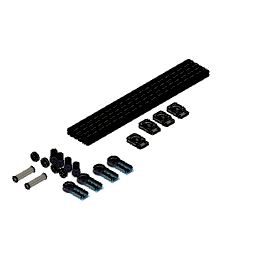
Conveyer Assemble v6 (Autodesk Fusion 360 design; units mm, degrees)
Autodesk Fusion 360 part; units mm, degrees
sketch "Sketch1" plane through (0, 0, 0) normal (0, 0, 1) x (1, 0, 0) in component "conveyerarm v2"
  line L0 (13.2288, 15) -> (80.2288, 15)
  line L1 (80.2288, 15) -> (80.2288, -15)
  line L2 (80.2288, -15) -> (13.2288, -15)
  arc A0 (13.2288, 15) -> (13.2288, -15) centre (0, 0) ccw
  dimension "d1" = 40
  dimension "d25" = 67
  constraint coincident A0.centre origin
  constraint horizontal L0
  constraint vertical L1
  constraint horizontal L2
  measures "d1" diameter of A0
  measures "d25" distance of L0.end L0.start
extrude "Extrude1" add sketch "Sketch1" along normal blind 14 makes body 1 in component "conveyerarm v2"
sketch "Sketch4" plane through (0, 0, 14) normal (0, 0, 1) x (-1, 0, 0) in component "conveyerarm v2"
  line L0 (-80.2288, -15) -> (-13.2288, -15)
  arc A0 (-13.2288, -15) -> (-13.2288, 15) centre (0, 0) ccw
  line L1 (-13.2288, 15) -> (-80.2288, 15)
  line L2 (-80.2288, 15) -> (-80.2288, -15)
  arc A1 (-12.49, -10) -> (-12.49, 10) centre (0, 0) ccw
  line L3 (-80.2288, -10) -> (-13.2288, -10)
  line L4 (-66, -10) -> (-12.49, -10)
  line L5 (-12.49, 10) -> (-80.2288, 10)
  dimension "d9" = -5
  constraint concentric A0 A1
  constraint coincident L2 L5.end
extrude "Extrude2" cut sketch "Sketch4" against normal blind 6.5 contours L2 A1 L3 L4 L5 bodies 1 in component "conveyerarm v2"
sketch "Sketch5" plane through (0, 0, 7.5) normal (0, 0, 1) x (-1, 0, 0) in component "conveyerarm v2"
  line L0 (-12.49, 10) -> (-80.2288, 10)
  line L1 (-80.2288, 10) -> (-80.2288, -10)
  line L2 (-80.2288, -10) -> (-12.49, -10)
  arc A0 (-12.49, -10) -> (-12.49, 10) centre (0, 0) ccw
  circle A1 centre (0, 0) radius 16
  dimension "d13" = 32
  constraint concentric A0 A1
  measures "d13" diameter of A1
extrude "Extrude3" cut sketch "Sketch5" against normal blind 3.5 contours A0 A1 bodies 1 in component "conveyerarm v2"
sketch "Sketch6" plane through (0, 0, 4) normal (0, 0, 1) x (-1, 0, 0) in component "conveyerarm v2"
  circle A0 centre (0, 0) radius 16
  circle A1 centre (0, 0) radius 12
  dimension "d16" = 24
  constraint coincident A0.centre A1.centre
  measures "d16" diameter of A1
extrude "Extrude4" cut sketch "Sketch6" against normal blind 5 contours A1 bodies 1 in component "conveyerarm v2"
sketch "Sketch7" plane through (0, 0, 7.5) normal (0, 0, 1) x (-1, 0, 0) in component "conveyerarm v2"
  arc A0 (-12.49, 10) -> (-12.49, -10) centre (0, 0) ccw
  line L0 (-12.49, 10) -> (-80.2288, 10)
  line L1 (-80.2288, 10) -> (-80.2288, -10)
  line L2 (-80.2288, -10) -> (-12.49, -10)
  circle A1 centre (-70.7288, 0) radius 2.6
  circle A2 centre (-48.7288, 0) radius 2.6
  circle A3 centre (-32.2288, 0) radius 2.6
  dimension "d20" = 5.2
  dimension "d21" = 22
  dimension "d22" = 5.2
  dimension "d23" = 16.5
  dimension "d24" = 5.2
  measures "d20" diameter of A1
  measures "d21" distance of A1.centre A2.centre
  measures "d22" diameter of A2
  measures "d23" distance of A2.centre A3.centre
  measures "d24" diameter of A3
extrude "Extrude5" cut sketch "Sketch7" against normal through all contours A1 | A2 | A3 bodies 1 in component "conveyerarm v2"
fillet "Fillet1" radius 5 2 edges at (80.2288, -15, 7) (80.2288, 15, 7) on bodies 1 in component "conveyerarm v2"
sketch "Sketch1 (2)" plane through (0, 0, 0) normal (0, 0, 1) x (1, 0, 0) in component "ConveyerLeg1 v3"
  line L0 (0, 0) -> (70, 0)
  line L1 (70, 0) -> (70, 42)
  line L2 (70, 42) -> (0, 42)
  line L3 (0, 42) -> (0, 0)
  dimension "d1_1" = 70
  dimension "d2" = 42
  constraint horizontal L0
  constraint vertical L1
  constraint horizontal L2
  constraint vertical L3
  constraint coincident L0.start L3.end
  measures "d1_1" distance of L1.end L2.end
  measures "d2" distance of L0.end L1.end
extrude "Extrude1'" add sketch "Sketch1 (2)" along normal blind 5 separate body makes body 2 in component "ConveyerLeg1 v3"
sketch "Sketch2" plane through (0, 0, 5) normal (0, 0, 1) x (-1, 0, 0) in component "ConveyerLeg1 v3"
  line L0 (0, -42) -> (0, 0)
  line L1 (0, 0) -> (-70, 0)
  line L2 (-70, 0) -> (-70, -42)
  line L3 (-70, -42) -> (0, -42)
  line L4 (0, 0) -> (-50, 0)
  line L5 (-50, 0) -> (-50, -42)
  line L6 (-50, -42) -> (0, -42)
  line L7 (0, -42) -> (0, 0)
  dimension "d5" = 50
  constraint horizontal L4
  constraint vertical L5
  constraint horizontal L6
  constraint vertical L7
  constraint coincident L0.end L1.start
  measures "d5" distance of L0.end L4.end
extrude "Extrude2'" add sketch "Sketch2" along normal blind 7.5 contours L0 L1 L3 L4 L5 L6 L7 bodies 2 in component "ConveyerLeg1 v3"
sketch "Sketch3" plane through (0, 0, 12.5) normal (0, 0, 1) x (-1, 0, 0) in component "ConveyerLeg1 v3"
  line L0 (0, -42) -> (0, 0)
  line L1 (0, 0) -> (-50, 0)
  line L2 (-50, 0) -> (-50, -42)
  line L3 (-50, -42) -> (0, -42)
  circle A0 centre (-25, -21) radius 18.75
  dimension "d8" = 37.5
  measures "d8" diameter of A0
hole "Hole1" at (25, 21, 12.5) direction (0, 0, -1) diameter 37.5 depth 10 tip angle 180 bodies 2 in component "ConveyerLeg1 v3"
sketch "Sketch7 (2)" plane through (0, 0, 12.5) normal (0, 0, 1) x (1, 0, 0) in component "ConveyerLeg1 v3"
  circle A0 centre (18, 21) radius 6.1
  circle A1 centre (11.3601, 28.875) radius 1.6
  circle A2 centre (25, 5.25) radius 1.6
  circle A3 centre (38.6399, 28.875) radius 1.6
  circle A4 centre (25, 36.75) radius 1.6
  circle A5 centre (25, 21) radius 18.75
  line L0 (0, 42) -> (0, 0)
  line L1 (0, 0) -> (50, 0)
  line L2 (50, 0) -> (50, 42)
  line L3 (50, 42) -> (0, 42)
  point P0 (25, 21)
  dimension "d16_1" = 3.2
  dimension "d17_1" = 3.2
  dimension "d18_1" = 3.2
  dimension "d19" = 3.2
  dimension "d41" = 12.2
  measures "d16_1" diameter of A1
  measures "d17_1" diameter of A2
  measures "d18_1" diameter of A3
  measures "d19" diameter of A4
  measures "d41" diameter of A0
extrude "Extrude3'" cut sketch "Sketch7 (2)" against normal through all contours A0 bodies 2 in component "ConveyerLeg1 v3"
extrude "Extrude4'" cut sketch "Sketch7 (2)" against normal through all contours A4 bodies 2 in component "ConveyerLeg1 v3"
extrude "Extrude5'" cut sketch "Sketch7 (2)" along normal through all and the other way through all contours A3 bodies 2 in component "ConveyerLeg1 v3"
extrude "Extrude6" cut sketch "Sketch7 (2)" along normal through all and the other way through all contours A2 bodies 2 in component "ConveyerLeg1 v3"
extrude "Extrude7" cut sketch "Sketch7 (2)" along normal through all and the other way through all contours A1 bodies 2 in component "ConveyerLeg1 v3"
sketch "Sketch9" plane through (0, 0, 5) normal (0, 0, 1) x (-1, 0, 0) in component "ConveyerLeg1 v3"
  circle A0 centre (-60, -35) radius 2.65
  circle A1 centre (-60, -7) radius 2.65
  dimension "d25_1" = 5.3
  dimension "d26_1" = 5.3
  measures "d25_1" diameter of A0
  measures "d26_1" diameter of A1
extrude "Extrude8" cut sketch "Sketch9" along normal mid plane 20 contours A0 bodies 2 in component "ConveyerLeg1 v3"
extrude "Extrude9" cut sketch "Sketch9" against normal blind 10 contours A1 bodies 2 in component "ConveyerLeg1 v3"
fillet "Fillet1'" radius 5 1 edges at (70, 42, 2.5) on bodies 2 in component "ConveyerLeg1 v3"
fillet "Fillet2" radius 5 1 edges at (70, 0, 2.5) on bodies 2 in component "ConveyerLeg1 v3"
fillet "Fillet3" radius 5 2 edges at (0, 0, 6.25) (0, 42, 6.25) on bodies 2 in component "ConveyerLeg1 v3"
sketch "Sketch10" plane through (0, 0, 12.5) normal (0, 0, 1) x (-1, 0, 0) in component "ConveyerLeg1 v3"
  circle A0 centre (-11.3598, -13.1248) radius 1.55
  circle A1 centre (-38.6402, -13.1248) radius 1.55
  point P0 (-25, -21)
  dimension "d37" = 3.1
  dimension "d38" = 3.1
  measures "d37" diameter of A0
  measures "d38" diameter of A1
extrude "Extrude10" cut sketch "Sketch10" along normal through all and the other way through all contours A1 bodies 2 in component "ConveyerLeg1 v3"
extrude "Extrude11" cut sketch "Sketch10" along normal through all and the other way through all contours A0 bodies 2 in component "ConveyerLeg1 v3"
sketch "Sketch11" plane through (0, 0, 0) normal (0, 0, 1) x (1, 0, 0) in component "ConveyerLeg1 v3"
sketch "Sketch1 (3)" plane through (0, 0, 0) normal (0, 0, 1) x (1, 0, 0) in component "CONVEYERROLLERv2 v4"
  circle A0 centre (0, 0) radius 9.95
  dimension "d1_3" = 19.9
  constraint coincident A0.centre origin
  measures "d1_3" diameter of A0
extrude "Extrude1''" add sketch "Sketch1 (3)" along normal blind 40 separate body makes body 3 in component "CONVEYERROLLERv2 v4"
sketch "Sketch2 (2)" plane through (0, 0, 0) normal (1, 0, 0) x (0, 1, 0) in component "CONVEYERROLLERv2 v4"
  line L0 (-12, 12) -> (-9.9, 9.9)
  line L1 (-12, 12) -> (-9.9, 14.1)
  line L2 (-9.9, 9.9) -> (-9.9, 14.1)
  constraint perpendicular L0 L1
revolve "Revolve1" add sketch "Sketch2 (2)" angle 360 about axis through (0, 0, 0) along (0, 0, -1) separate body makes body 4 in component "CONVEYERROLLERv2 v4"
sketch "Sketch4 (2)" plane through (0, 0, 40) normal (0, 0, 1) x (-1, 0, 0) in component "CONVEYERROLLERv2 v4"
  line L0 (-9.4994, -0.1031) -> (-9.4994, -0.1031)
  circle A0 centre (0, 0) radius 8.5
  circle A1 centre (0, 0) radius 10
  dimension "d32_2" = 17
  dimension "d33_2" = 20
  constraint coincident A0.centre A1.centre
  constraint concentric A0 A1
  measures "d32_2" diameter of A0
  measures "d33_2" diameter of A1
extrude "Extrude6'" cut sketch "Sketch4 (2)" against normal blind 18 bodies 3 in component "CONVEYERROLLERv2 v4"
sketch "Sketch9 (2)" plane through (0, 0, 40) normal (0, 0, 1) x (-1, 0, 0) in component "CONVEYERROLLERv2 v4"
  circle A0 centre (0, 0) radius 8.5
  line L0 (7.1105, -6.3018) -> (6.4494, -5.5367)
  line L1 (5.8562, -6.1607) -> (6.6539, -6.7822)
  line L2 (7.1105, -6.3018) -> (6.6539, -6.7822)
  line L3 (5.8562, -6.1607) -> (6.4494, -5.5367)
  line L4 (6.9765, -4.8558) -> (7.8829, -5.3039)
  line L5 (8.2335, -4.7415) -> (7.8829, -5.3039)
  line L6 (8.2335, -4.7415) -> (7.4319, -4.1251)
  line L7 (6.9765, -4.8558) -> (7.4319, -4.1251)
  line L8 (7.8111, -3.352) -> (8.7892, -3.6085)
  line L9 (9.0194, -2.9871) -> (8.7892, -3.6085)
  line L10 (9.0194, -2.9871) -> (8.1102, -2.5446)
  line L11 (7.8111, -3.352) -> (8.1102, -2.5446)
  line L12 (8.326, -1.711) -> (9.3357, -1.7654)
  line L13 (9.4361, -1.1103) -> (9.3357, -1.7654)
  line L14 (9.4361, -1.1103) -> (8.4564, -0.8599)
  line L15 (8.326, -1.711) -> (8.4564, -0.8599)
  line L16 (8.5, 0) -> (9.5, 0.15)
  line L17 (9.4664, 0.8119) -> (9.5, 0.15)
  line L18 (9.4664, 0.8119) -> (8.4564, 0.8599)
  line L19 (8.5, 0) -> (8.4564, 0.8599)
  line L20 (8.326, 1.711) -> (9.2753, 2.0593)
  line L21 (9.1092, 2.7008) -> (9.2753, 2.0593)
  line L22 (9.1092, 2.7008) -> (8.1102, 2.5446)
  line L23 (8.326, 1.711) -> (8.1102, 2.5446)
  line L24 (7.8111, 3.352) -> (8.6709, 3.8842)
  line L25 (8.3791, 4.4792) -> (8.6709, 3.8842)
  line L26 (8.3791, 4.4792) -> (7.4319, 4.1251)
  line L27 (7.8111, 3.352) -> (7.4319, 4.1251)
  line L28 (6.9765, 4.8558) -> (7.7116, 5.5502)
  line L29 (7.3059, 6.0742) -> (7.7116, 5.5502)
  line L30 (7.3059, 6.0742) -> (6.4494, 5.5367)
  line L31 (6.9765, 4.8558) -> (6.4494, 5.5367)
  line L32 (5.8562, 6.1607) -> (6.4365, 6.9889)
  line L33 (5.9336, 7.4206) -> (6.4365, 6.9889)
  line L34 (5.9336, 7.4206) -> (5.2029, 6.7216)
  line L35 (5.8562, 6.1607) -> (5.2029, 6.7216)
  line L36 (4.4962, 7.2135) -> (4.8979, 8.1415)
  line L37 (4.3184, 8.4631) -> (4.8979, 8.1415)
  line L38 (4.3184, 8.4631) -> (3.7434, 7.6313)
  line L39 (4.4962, 7.2135) -> (3.7434, 7.6313)
  line L40 (2.9521, 7.9709) -> (3.1587, 8.9607)
  line L41 (2.5264, 9.1591) -> (3.1587, 8.9607)
  line L42 (2.5264, 9.1591) -> (2.1305, 8.2287)
  line L43 (2.9521, 7.9709) -> (2.1305, 8.2287)
  line L44 (1.2871, 8.402) -> (1.2903, 9.4132)
  line L45 (0.631, 9.4802) -> (1.2903, 9.4132)
  line L46 (0.631, 9.4802) -> (0.4305, 8.4891)
  line L47 (1.2871, 8.402) -> (0.4305, 8.4891)
  line L48 (-0.4305, 8.4891) -> (-0.631, 9.4802)
  line L49 (-1.2903, 9.4132) -> (-0.631, 9.4802)
  line L50 (-1.2903, 9.4132) -> (-1.2871, 8.402)
  line L51 (-0.4305, 8.4891) -> (-1.2871, 8.402)
  line L52 (-2.1305, 8.2287) -> (-2.5264, 9.1591)
  line L53 (-3.1587, 8.9607) -> (-2.5264, 9.1591)
  line L54 (-3.1587, 8.9607) -> (-2.9521, 7.9709)
  line L55 (-2.1305, 8.2287) -> (-2.9521, 7.9709)
  line L56 (-3.7434, 7.6313) -> (-4.3184, 8.4631)
  line L57 (-4.8979, 8.1415) -> (-4.3184, 8.4631)
  line L58 (-4.8979, 8.1415) -> (-4.4962, 7.2135)
  line L59 (-3.7434, 7.6313) -> (-4.4962, 7.2135)
  line L60 (-5.2029, 6.7216) -> (-5.9336, 7.4206)
  line L61 (-6.4365, 6.9889) -> (-5.9336, 7.4206)
  line L62 (-6.4365, 6.9889) -> (-5.8562, 6.1607)
  line L63 (-5.2029, 6.7216) -> (-5.8562, 6.1607)
  line L64 (-6.4494, 5.5367) -> (-7.3059, 6.0742)
  line L65 (-7.7116, 5.5502) -> (-7.3059, 6.0742)
  line L66 (-7.7116, 5.5502) -> (-6.9765, 4.8558)
  line L67 (-6.4494, 5.5367) -> (-6.9765, 4.8558)
  line L68 (-7.4319, 4.1251) -> (-8.3791, 4.4792)
  line L69 (-8.6709, 3.8842) -> (-8.3791, 4.4792)
  line L70 (-8.6709, 3.8842) -> (-7.8111, 3.352)
  line L71 (-7.4319, 4.1251) -> (-7.8111, 3.352)
  line L72 (-8.1102, 2.5446) -> (-9.1092, 2.7008)
  line L73 (-9.2753, 2.0593) -> (-9.1092, 2.7008)
  line L74 (-9.2753, 2.0593) -> (-8.326, 1.711)
  line L75 (-8.1102, 2.5446) -> (-8.326, 1.711)
  line L76 (-8.4564, 0.8599) -> (-9.4664, 0.8119)
  line L77 (-9.5, 0.15) -> (-9.4664, 0.8119)
  line L78 (-9.5, 0.15) -> (-8.5, 0)
  line L79 (-8.4564, 0.8599) -> (-8.5, 0)
  line L80 (-8.4564, -0.8599) -> (-9.4361, -1.1103)
  line L81 (-9.3357, -1.7654) -> (-9.4361, -1.1103)
  line L82 (-9.3357, -1.7654) -> (-8.326, -1.711)
  line L83 (-8.4564, -0.8599) -> (-8.326, -1.711)
  line L84 (-8.1102, -2.5446) -> (-9.0194, -2.9871)
  line L85 (-8.7892, -3.6085) -> (-9.0194, -2.9871)
  line L86 (-8.7892, -3.6085) -> (-7.8111, -3.352)
  line L87 (-8.1102, -2.5446) -> (-7.8111, -3.352)
  line L88 (-7.4319, -4.1251) -> (-8.2335, -4.7415)
  line L89 (-7.8829, -5.3039) -> (-8.2335, -4.7415)
  line L90 (-7.8829, -5.3039) -> (-6.9765, -4.8558)
  line L91 (-7.4319, -4.1251) -> (-6.9765, -4.8558)
  line L92 (-6.4494, -5.5367) -> (-7.1105, -6.3018)
  line L93 (-6.6539, -6.7822) -> (-7.1105, -6.3018)
  line L94 (-6.6539, -6.7822) -> (-5.8562, -6.1607)
  line L95 (-6.4494, -5.5367) -> (-5.8562, -6.1607)
  line L96 (-5.2029, -6.7216) -> (-5.6964, -7.6042)
  line L97 (-5.1524, -7.9828) -> (-5.6964, -7.6042)
  line L98 (-5.1524, -7.9828) -> (-4.4962, -7.2135)
  line L99 (-5.2029, -6.7216) -> (-4.4962, -7.2135)
  line L100 (-3.7434, -7.6313) -> (-4.0491, -8.5952)
  line L101 (-3.4401, -8.8566) -> (-4.0491, -8.5952)
  line L102 (-3.4401, -8.8566) -> (-2.9521, -7.9709)
  line L103 (-3.7434, -7.6313) -> (-2.9521, -7.9709)
  line L104 (-2.1305, -8.2287) -> (-2.236, -9.2343)
  line L105 (-1.5868, -9.3677) -> (-2.236, -9.2343)
  line L106 (-1.5868, -9.3677) -> (-1.2871, -8.402)
  line L107 (-2.1305, -8.2287) -> (-1.2871, -8.402)
  line L108 (-0.4305, -8.4891) -> (-0.3314, -9.4954)
  line L109 (0.3314, -9.4954) -> (-0.3314, -9.4954)
  line L110 (0.3314, -9.4954) -> (0.4305, -8.4891)
  line L111 (-0.4305, -8.4891) -> (0.4305, -8.4891)
  line L112 (1.2871, -8.402) -> (1.5868, -9.3677)
  line L113 (2.236, -9.2343) -> (1.5868, -9.3677)
  line L114 (2.236, -9.2343) -> (2.1305, -8.2287)
  line L115 (1.2871, -8.402) -> (2.1305, -8.2287)
  line L116 (2.9521, -7.9709) -> (3.4401, -8.8566)
  line L117 (4.0491, -8.5952) -> (3.4401, -8.8566)
  line L118 (4.0491, -8.5952) -> (3.7434, -7.6313)
  line L119 (2.9521, -7.9709) -> (3.7434, -7.6313)
  line L120 (4.4962, -7.2135) -> (5.1524, -7.9828)
  line L121 (5.6964, -7.6042) -> (5.1524, -7.9828)
  line L122 (5.6964, -7.6042) -> (5.2029, -6.7216)
  line L123 (4.4962, -7.2135) -> (5.2029, -6.7216)
  dimension "d42_1" = 360
extrude "Extrude7'" add sketch "Sketch9 (2)" against normal blind 18 contours A0 L16 L17 L18 | A0 L12 L13 L14 | A0 L20 L21 L22 | A0 L8 L9 L10 | A0 L24 L25 L26 | A0 L4 L5 L6 | A0 L28 L29 L30 | A0 L0 L1 L2 | A0 L32 L33 L34 | A0 L120 L121 L122 | A0 L36 L37 L38 | A0 L116 L117 L118 | A0 L40 L41 L42 | A0 L112 L113 L114 | A0 L44 L45 L46 | A0 L108 L109 L110 | A0 L48 L49 L50 | A0 L104 L105 L106 | A0 L52 L53 L54 | A0 L100 L101 L102 | A0 L56 L57 L58 | A0 L96 L97 L98 | A0 L60 L61 L62 | A0 L92 L93 L94 | A0 L64 L65 L66 | A0 L88 L89 L90 | A0 L68 L69 L70 | A0 L84 L85 L86 | A0 L72 L73 L74 | A0 L80 L81 L82 | A0 L76 L77 L78 bodies 3 in component "CONVEYERROLLERv2 v4"
sketch "Sketch11 (2)" plane through (0, 0, 40) normal (0, 0, 1) x (-1, 0, 0) in component "CONVEYERROLLERv2 v4"
  arc A0 (-4.4962, -7.2135) -> (-3.7434, -7.6313) centre (0, 0) ccw
  line L0 (-3.7434, -7.6313) -> (-4.0491, -8.5952)
  line L1 (-4.0491, -8.5952) -> (-3.4401, -8.8566)
  line L2 (-3.4401, -8.8566) -> (-2.9521, -7.9709)
  arc A1 (-2.9521, -7.9709) -> (-2.1305, -8.2287) centre (0, 0) ccw
  line L3 (-2.1305, -8.2287) -> (-2.236, -9.2343)
  line L4 (-2.236, -9.2343) -> (-1.5868, -9.3677)
  line L5 (-1.5868, -9.3677) -> (-1.2871, -8.402)
  arc A2 (-1.2871, -8.402) -> (-0.4305, -8.4891) centre (0, 0) ccw
  line L6 (-0.4305, -8.4891) -> (-0.3314, -9.4954)
  line L7 (-0.3314, -9.4954) -> (0.3314, -9.4954)
  line L8 (0.3314, -9.4954) -> (0.4305, -8.4891)
  arc A3 (0.4305, -8.4891) -> (1.2871, -8.402) centre (0, 0) ccw
  line L9 (1.2871, -8.402) -> (1.5868, -9.3677)
  line L10 (1.5868, -9.3677) -> (2.236, -9.2343)
  line L11 (2.236, -9.2343) -> (2.1305, -8.2287)
  arc A4 (2.1305, -8.2287) -> (2.9521, -7.9709) centre (0, 0) ccw
  line L12 (2.9521, -7.9709) -> (3.4401, -8.8566)
  line L13 (3.4401, -8.8566) -> (4.0491, -8.5952)
  line L14 (4.0491, -8.5952) -> (3.7434, -7.6313)
  arc A5 (3.7434, -7.6313) -> (4.4962, -7.2135) centre (0, 0) ccw
  line L15 (4.4962, -7.2135) -> (5.1524, -7.9828)
  line L16 (5.1524, -7.9828) -> (5.6964, -7.6042)
  line L17 (5.6964, -7.6042) -> (5.2029, -6.7216)
  arc A6 (5.2029, -6.7216) -> (5.8562, -6.1607) centre (0, 0) ccw
  line L18 (5.8562, -6.1607) -> (6.6539, -6.7822)
  line L19 (6.6539, -6.7822) -> (7.1105, -6.3018)
  line L20 (7.1105, -6.3018) -> (6.4494, -5.5367)
  arc A7 (6.4494, -5.5367) -> (6.9765, -4.8558) centre (0, 0) ccw
  line L21 (6.9765, -4.8558) -> (7.8829, -5.3039)
  line L22 (7.8829, -5.3039) -> (8.2335, -4.7415)
  line L23 (8.2335, -4.7415) -> (7.4319, -4.1251)
  arc A8 (7.4319, -4.1251) -> (7.8111, -3.352) centre (0, 0) ccw
  line L24 (7.8111, -3.352) -> (8.7892, -3.6085)
  line L25 (8.7892, -3.6085) -> (9.0194, -2.9871)
  line L26 (9.0194, -2.9871) -> (8.1102, -2.5446)
  arc A9 (8.1102, -2.5446) -> (8.326, -1.711) centre (0, 0) ccw
  line L27 (8.326, -1.711) -> (9.3357, -1.7654)
  line L28 (9.3357, -1.7654) -> (9.4361, -1.1103)
  line L29 (9.4361, -1.1103) -> (8.4564, -0.8599)
  arc A10 (8.4564, -0.8599) -> (8.5, 0) centre (0, 0) ccw
  line L30 (8.5, 0) -> (9.5, 0.15)
  line L31 (9.5, 0.15) -> (9.4664, 0.8119)
  line L32 (9.4664, 0.8119) -> (8.4564, 0.8599)
  arc A11 (8.4564, 0.8599) -> (8.326, 1.711) centre (0, 0) ccw
  line L33 (8.326, 1.711) -> (9.2753, 2.0593)
  line L34 (9.2753, 2.0593) -> (9.1092, 2.7008)
  line L35 (9.1092, 2.7008) -> (8.1102, 2.5446)
  arc A12 (8.1102, 2.5446) -> (7.8111, 3.352) centre (0, 0) ccw
  line L36 (7.8111, 3.352) -> (8.6709, 3.8842)
  line L37 (8.6709, 3.8842) -> (8.3791, 4.4792)
  line L38 (8.3791, 4.4792) -> (7.4319, 4.1251)
  arc A13 (7.4319, 4.1251) -> (6.9765, 4.8558) centre (0, 0) ccw
  line L39 (6.9765, 4.8558) -> (7.7116, 5.5502)
  line L40 (7.7116, 5.5502) -> (7.3059, 6.0742)
  line L41 (7.3059, 6.0742) -> (6.4494, 5.5367)
  arc A14 (6.4494, 5.5367) -> (5.8562, 6.1607) centre (0, 0) ccw
  line L42 (5.8562, 6.1607) -> (6.4365, 6.9889)
  line L43 (6.4365, 6.9889) -> (5.9336, 7.4206)
  line L44 (5.9336, 7.4206) -> (5.2029, 6.7216)
  arc A15 (5.2029, 6.7216) -> (4.4962, 7.2135) centre (0, 0) ccw
  line L45 (4.4962, 7.2135) -> (4.8979, 8.1415)
  line L46 (4.8979, 8.1415) -> (4.3184, 8.4631)
  line L47 (4.3184, 8.4631) -> (3.7434, 7.6313)
  arc A16 (3.7434, 7.6313) -> (2.9521, 7.9709) centre (0, 0) ccw
  line L48 (2.9521, 7.9709) -> (3.1587, 8.9607)
  line L49 (3.1587, 8.9607) -> (2.5264, 9.1591)
  line L50 (2.5264, 9.1591) -> (2.1305, 8.2287)
  arc A17 (2.1305, 8.2287) -> (1.2871, 8.402) centre (0, 0) ccw
  line L51 (1.2871, 8.402) -> (1.2903, 9.4132)
  line L52 (1.2903, 9.4132) -> (0.631, 9.4802)
  line L53 (0.631, 9.4802) -> (0.4305, 8.4891)
  arc A18 (0.4305, 8.4891) -> (-0.4305, 8.4891) centre (0, 0) ccw
  line L54 (-0.4305, 8.4891) -> (-0.631, 9.4802)
  line L55 (-0.631, 9.4802) -> (-1.2903, 9.4132)
  line L56 (-1.2903, 9.4132) -> (-1.2871, 8.402)
  arc A19 (-1.2871, 8.402) -> (-2.1305, 8.2287) centre (0, 0) ccw
  line L57 (-2.1305, 8.2287) -> (-2.5264, 9.1591)
  line L58 (-2.5264, 9.1591) -> (-3.1587, 8.9607)
  line L59 (-3.1587, 8.9607) -> (-2.9521, 7.9709)
  arc A20 (-2.9521, 7.9709) -> (-3.7434, 7.6313) centre (0, 0) ccw
  line L60 (-3.7434, 7.6313) -> (-4.3184, 8.4631)
  line L61 (-4.3184, 8.4631) -> (-4.8979, 8.1415)
  line L62 (-4.8979, 8.1415) -> (-4.4962, 7.2135)
  arc A21 (-4.4962, 7.2135) -> (-5.2029, 6.7216) centre (0, 0) ccw
  line L63 (-5.2029, 6.7216) -> (-5.9336, 7.4206)
  line L64 (-5.9336, 7.4206) -> (-6.4365, 6.9889)
  line L65 (-6.4365, 6.9889) -> (-5.8562, 6.1607)
  arc A22 (-5.8562, 6.1607) -> (-6.4494, 5.5367) centre (0, 0) ccw
  line L66 (-6.4494, 5.5367) -> (-7.3059, 6.0742)
  line L67 (-7.3059, 6.0742) -> (-7.7116, 5.5502)
  line L68 (-7.7116, 5.5502) -> (-6.9765, 4.8558)
  arc A23 (-6.9765, 4.8558) -> (-7.4319, 4.1251) centre (0, 0) ccw
  line L69 (-7.4319, 4.1251) -> (-8.3791, 4.4792)
  line L70 (-8.3791, 4.4792) -> (-8.6709, 3.8842)
  line L71 (-8.6709, 3.8842) -> (-7.8111, 3.352)
  arc A24 (-7.8111, 3.352) -> (-8.1102, 2.5446) centre (0, 0) ccw
  line L72 (-8.1102, 2.5446) -> (-9.1092, 2.7008)
  line L73 (-9.1092, 2.7008) -> (-9.2753, 2.0593)
  line L74 (-9.2753, 2.0593) -> (-8.326, 1.711)
  arc A25 (-8.326, 1.711) -> (-8.4564, 0.8599) centre (0, 0) ccw
  line L75 (-8.4564, 0.8599) -> (-9.4664, 0.8119)
  line L76 (-9.4664, 0.8119) -> (-9.5, 0.15)
  line L77 (-9.5, 0.15) -> (-8.5, 0)
  arc A26 (-8.5, 0) -> (-8.4564, -0.8599) centre (0, 0) ccw
  line L78 (-8.4564, -0.8599) -> (-9.4361, -1.1103)
  line L79 (-9.4361, -1.1103) -> (-9.3357, -1.7654)
  line L80 (-9.3357, -1.7654) -> (-8.326, -1.711)
  arc A27 (-8.326, -1.711) -> (-8.1102, -2.5446) centre (0, 0) ccw
  line L81 (-8.1102, -2.5446) -> (-9.0194, -2.9871)
  line L82 (-9.0194, -2.9871) -> (-8.7892, -3.6085)
  line L83 (-8.7892, -3.6085) -> (-7.8111, -3.352)
  arc A28 (-7.8111, -3.352) -> (-7.4319, -4.1251) centre (0, 0) ccw
  line L84 (-7.4319, -4.1251) -> (-8.2335, -4.7415)
  line L85 (-8.2335, -4.7415) -> (-7.8829, -5.3039)
  line L86 (-7.8829, -5.3039) -> (-6.9765, -4.8558)
  arc A29 (-6.9765, -4.8558) -> (-6.4494, -5.5367) centre (0, 0) ccw
  line L87 (-6.4494, -5.5367) -> (-7.1105, -6.3018)
  line L88 (-7.1105, -6.3018) -> (-6.6539, -6.7822)
  line L89 (-6.6539, -6.7822) -> (-5.8562, -6.1607)
  arc A30 (-5.8562, -6.1607) -> (-5.2029, -6.7216) centre (0, 0) ccw
  line L90 (-5.2029, -6.7216) -> (-5.6964, -7.6042)
  line L91 (-5.6964, -7.6042) -> (-5.1524, -7.9828)
  line L92 (-5.1524, -7.9828) -> (-4.4962, -7.2135)
  circle A31 centre (0, 0) radius 4
  dimension "d45_1" = 8
  constraint concentric A0 A31
  measures "d45_1" diameter of A31
extrude "Extrude8'" cut sketch "Sketch11 (2)" against normal through all contours A31 bodies 3 in component "CONVEYERROLLERv2 v4"
fillet "Fillet1''" radius 0.1 2 edges at (4.3184, -8.4631, 31) (4.8979, -8.1415, 31) on bodies 3 in component "CONVEYERROLLERv2 v4"
fillet "Fillet2'" radius 0.1 9 edges at (3.1587, -8.9607, 31) (2.5264, -9.1591, 31) (1.2903, -9.4132, 31) (0.631, -9.4802, 31) (-0.631, -9.4802, 31) (6.4365, -6.9889, 31) (5.9336, -7.4206, 31) (7.3059, -6.0742, 31) (7.7116, -5.5502, 31) on bodies 3 in component "CONVEYERROLLERv2 v4"
fillet "Fillet3'" radius 0.1 51 edges at (8.3791, -4.4792, 31) (8.6709, -3.8842, 31) (9.1092, -2.7008, 31) (9.2753, -2.0593, 31) (9.4664, -0.8119, 31) (9.5, -0.15, 31) (9.4361, 1.1103, 31) (9.3357, 1.7654, 31) (9.0194, 2.9871, 31) (8.7892, 3.6085, 31) (8.2335, 4.7415, 31) (7.8829, 5.3039, 31) (7.1105, 6.3018, 31) (6.6539, 6.7822, 31) (5.6964, 7.6042, 31) (-9.3357, 1.7654, 31) (-9.4361, 1.1103, 31) (-9.5, -0.15, 31) (-9.4664, -0.8119, 31) (-9.2753, -2.0593, 31) (-9.1092, -2.7008, 31) (-8.6709, -3.8842, 31) (-8.3791, -4.4792, 31) (-7.7116, -5.5502, 31) (-7.3059, -6.0742, 31) (-6.4365, -6.9889, 31) (-5.9336, -7.4206, 31) (-4.8979, -8.1415, 31) (-4.3184, -8.4631, 31) (-3.1587, -8.9607, 31) (-2.5264, -9.1591, 31) (-1.2903, -9.4132, 31) (-9.0194, 2.9871, 31) (-8.7892, 3.6085, 31) (-8.2335, 4.7415, 31) (-7.8829, 5.3039, 31) (-7.1105, 6.3018, 31) (-6.6539, 6.7822, 31) (-5.6964, 7.6042, 31) (-5.1524, 7.9828, 31) (-4.0491, 8.5952, 31) (-2.236, 9.2343, 31) (-1.5868, 9.3677, 31) (-0.3314, 9.4954, 31) (0.3314, 9.4954, 31) (1.5868, 9.3677, 31) (2.236, 9.2343, 31) (3.4401, 8.8566, 31) (4.0491, 8.5952, 31) (5.1524, 7.9828, 31) (-3.4401, 8.8566, 31) on bodies 3 in component "CONVEYERROLLERv2 v4"
sketch "Sketch12" plane through (0, 0, 0) normal (0, 0, 1) x (1, 0, 0) in component "CONVEYERROLLERv2 v4"
  circle A0 centre (0, 0) radius 10.5
  circle A1 centre (0, 0) radius 8.85
  dimension "d54" = 21
  dimension "d55" = 17.7
  constraint coincident A0.centre A1.centre
  constraint concentric A0 A1
  measures "d54" diameter of A0
  measures "d55" diameter of A1
extrude "Extrude9'" cut sketch "Sketch12" along normal blind 9 bodies 3 in component "CONVEYERROLLERv2 v4"
combine "Combine4" operation add target body 3 tool bodies 4 in component "CONVEYERROLLERv2 v4"
sketch "Sketch1 (4)" plane through (0, 0, 0) normal (0, 1, 0) x (1, 0, 0) in component "ProfileBase"
  line L0 (0, 0) -> (100, 0)
  line L1 (100, 0) -> (100, -20)
  line L2 (100, -20) -> (0, -20)
  line L3 (0, -20) -> (0, 0)
  dimension "d53" = 100
  dimension "d58" = 20
  constraint horizontal L0
  constraint vertical L1
  constraint horizontal L2
  constraint vertical L3
  constraint coincident L0.start L3.end
  measures "d53" distance of L0.start L0.end
  measures "d58" distance of L0.start L2.end
extrude "Extrude1'''" add sketch "Sketch1 (4)" along normal blind 600 separate body makes body 5 in component "ProfileBase"
sketch "Sketch2 (3)" plane through (0, 0, 0) normal (0, -1, 0) x (1, 0, 0) in component "ProfileBase"
  line L0 (100, 20) -> (0, 20)
  line L1 (0, 20) -> (0, 0)
  line L2 (0, 0) -> (100, 0)
  line L3 (100, 0) -> (100, 20)
  circle A0 centre (10, 10) radius 2.5
  line L4 (0, 13) -> (2, 13)
  line L5 (2, 13) -> (2, 17)
  line L6 (2, 17) -> (6, 13)
  line L7 (6, 13) -> (6, 7)
  line L8 (6, 7) -> (2, 3)
  line L9 (2, 3) -> (2, 7)
  line L10 (2, 7) -> (0, 7)
  line L11 (0, 13) -> (0, 7)
  line L12 (3, 2) -> (7, 6)
  line L13 (7, 2) -> (3, 2)
  line L14 (7, 0) -> (7, 2)
  line L15 (7, 0) -> (13, 0)
  line L16 (13, 2) -> (13, 0)
  line L17 (17, 2) -> (13, 2)
  line L18 (13, 6) -> (17, 2)
  line L19 (7, 6) -> (13, 6)
  line L20 (18, 3) -> (14, 7)
  line L21 (18, 7) -> (18, 3)
  line L22 (20, 7) -> (18, 7)
  line L23 (20, 7) -> (20, 13)
  line L24 (18, 13) -> (20, 13)
  line L25 (18, 17) -> (18, 13)
  line L26 (14, 13) -> (18, 17)
  line L27 (14, 7) -> (14, 13)
  line L28 (17, 18) -> (13, 14)
  line L29 (13, 18) -> (17, 18)
  line L30 (13, 20) -> (13, 18)
  line L31 (13, 20) -> (7, 20)
  line L32 (7, 18) -> (7, 20)
  line L33 (3, 18) -> (7, 18)
  line L34 (7, 14) -> (3, 18)
  line L35 (13, 14) -> (7, 14)
  point P0 (6, 10)
  dimension "d61" = 5
  dimension "d62" = 10
  dimension "d63" = 10
  dimension "d64" = 4
  dimension "d65" = 6
  dimension "d66" = 2
  dimension "d67" = 2
  dimension "d69" = 3
  dimension "d70" = 6
  dimension "d71" = 3
  dimension "d72" = 90
  dimension "d74" = 360
  constraint coincident L1 L4.start
  constraint perpendicular L1 L4
  constraint perpendicular L4 L5
  constraint parallel L1 L7
  constraint parallel L7 L9
  constraint coincident L1 L10.end
  constraint perpendicular L1 L10
  constraint equal L5 L9
  constraint midpoint L7 P0
  measures "d61" diameter of A0
  measures "d62" distance of L1 A0.centre
  measures "d63" distance of L2 A0.centre
  measures "d64" distance of A0.centre L7
  measures "d65" distance of L6.end L7.end
  measures "d66" distance of L1 L5
  measures "d67" distance of L1 L9
  measures "d69" distance of A0.centre L10
  measures "d70" distance of L4 L10
  measures "d71" distance of L10 P0
  measures "d72" angle of L6 L8
extrude "Extrude2''" cut sketch "Sketch2 (3)" against normal through all contours L0 L28 L29 L30 L31 L32 L33 L34 L35 | L2 L12 L13 L14 L15 L16 L17 L18 L19 | L1 L4 L5 L6 L7 L8 L9 L10 L11 | A0 | L20 L21 L22 L23 L24 L25 L26 L27 bodies 5 in component "ProfileBase"
pattern_linear "R-Pattern1" count 5 spacing 20 along (1, 0, 0) of "Extrude2''" in component "ProfileBase"
sketch "Sketch3 (2)" plane through (0, 0, 0) normal (0, -1, 0) x (1, 0, 0) in component "ProfileBase"
  circle A0 centre (90, 10) radius 2.5
  line L0 (78, 13) -> (82, 13)
  line L1 (82, 13) -> (82, 17)
  line L2 (82, 17) -> (86, 13)
  line L3 (86, 13) -> (86, 7)
  line L4 (86, 7) -> (82, 3)
  line L5 (82, 3) -> (82, 7)
  line L6 (82, 7) -> (78, 7)
  line L7 (78, 7) -> (78, 3)
  line L8 (78, 3) -> (74, 7)
  line L9 (74, 7) -> (74, 13)
  line L10 (74, 13) -> (78, 17)
  line L11 (78, 17) -> (78, 13)
  circle A1 centre (70, 10) radius 2.5
  line L12 (58, 13) -> (62, 13)
  line L13 (62, 13) -> (62, 17)
  line L14 (62, 17) -> (66, 13)
  line L15 (66, 13) -> (66, 7)
  line L16 (66, 7) -> (62, 3)
  line L17 (62, 3) -> (62, 7)
  line L18 (62, 7) -> (58, 7)
  line L19 (58, 7) -> (58, 3)
  line L20 (58, 3) -> (54, 7)
  line L21 (54, 7) -> (54, 13)
  line L22 (54, 13) -> (58, 17)
  line L23 (58, 17) -> (58, 13)
  circle A2 centre (50, 10) radius 2.5
  line L24 (38, 13) -> (42, 13)
  line L25 (42, 13) -> (42, 17)
  line L26 (42, 17) -> (46, 13)
  line L27 (46, 13) -> (46, 7)
  line L28 (46, 7) -> (42, 3)
  line L29 (42, 3) -> (42, 7)
  line L30 (42, 7) -> (38, 7)
  line L31 (38, 7) -> (38, 3)
  line L32 (38, 3) -> (34, 7)
  line L33 (34, 7) -> (34, 13)
  line L34 (34, 13) -> (38, 17)
  line L35 (38, 17) -> (38, 13)
  circle A3 centre (30, 10) radius 2.5
  line L36 (100, 7) -> (98, 7)
  line L37 (98, 7) -> (98, 3)
  line L38 (98, 3) -> (94, 7)
  line L39 (94, 7) -> (94, 13)
  line L40 (94, 13) -> (98, 17)
  line L41 (98, 17) -> (98, 13)
  line L42 (98, 13) -> (100, 13)
  line L43 (100, 13) -> (100, 20)
  line L44 (100, 20) -> (93, 20)
  line L45 (93, 20) -> (93, 18)
  line L46 (93, 18) -> (97, 18)
  line L47 (97, 18) -> (93, 14)
  line L48 (93, 14) -> (87, 14)
  line L49 (87, 14) -> (83, 18)
  line L50 (83, 18) -> (87, 18)
  line L51 (87, 18) -> (87, 20)
  line L52 (87, 20) -> (73, 20)
  line L53 (73, 20) -> (73, 18)
  line L54 (73, 18) -> (77, 18)
  line L55 (77, 18) -> (73, 14)
  line L56 (73, 14) -> (67, 14)
  line L57 (67, 14) -> (63, 18)
  line L58 (63, 18) -> (67, 18)
  line L59 (67, 18) -> (67, 20)
  line L60 (67, 20) -> (53, 20)
  line L61 (53, 20) -> (53, 18)
  line L62 (53, 18) -> (57, 18)
  line L63 (57, 18) -> (53, 14)
  line L64 (53, 14) -> (47, 14)
  line L65 (47, 14) -> (43, 18)
  line L66 (43, 18) -> (47, 18)
  line L67 (47, 18) -> (47, 20)
  line L68 (47, 20) -> (33, 20)
  line L69 (33, 20) -> (33, 18)
  line L70 (33, 18) -> (37, 18)
  line L71 (37, 18) -> (33, 14)
  line L72 (33, 14) -> (27, 14)
  line L73 (27, 14) -> (23, 18)
  line L74 (23, 18) -> (27, 18)
  line L75 (27, 18) -> (27, 20)
  line L76 (27, 20) -> (13, 20)
  line L77 (13, 20) -> (13, 18)
  line L78 (13, 18) -> (17, 18)
  line L79 (17, 18) -> (13, 14)
  line L80 (13, 14) -> (7, 14)
  line L81 (7, 14) -> (3, 18)
  line L82 (3, 18) -> (7, 18)
  line L83 (7, 18) -> (7, 20)
  line L84 (7, 20) -> (0, 20)
  line L85 (0, 20) -> (0, 13)
  line L86 (0, 13) -> (2, 13)
  line L87 (2, 13) -> (2, 17)
  line L88 (2, 17) -> (6, 13)
  line L89 (6, 13) -> (6, 7)
  line L90 (6, 7) -> (2, 3)
  line L91 (2, 3) -> (2, 7)
  line L92 (2, 7) -> (0, 7)
  line L93 (0, 7) -> (0, 0)
  line L94 (0, 0) -> (7, 0)
  line L95 (7, 0) -> (7, 2)
  line L96 (7, 2) -> (3, 2)
  line L97 (3, 2) -> (7, 6)
  line L98 (7, 6) -> (13, 6)
  line L99 (13, 6) -> (17, 2)
  line L100 (17, 2) -> (13, 2)
  line L101 (13, 2) -> (13, 0)
  line L102 (13, 0) -> (27, 0)
  line L103 (27, 0) -> (27, 2)
  line L104 (27, 2) -> (23, 2)
  line L105 (23, 2) -> (27, 6)
  line L106 (27, 6) -> (33, 6)
  line L107 (33, 6) -> (37, 2)
  line L108 (37, 2) -> (33, 2)
  line L109 (33, 2) -> (33, 0)
  line L110 (33, 0) -> (47, 0)
  line L111 (47, 0) -> (47, 2)
  line L112 (47, 2) -> (43, 2)
  line L113 (43, 2) -> (47, 6)
  line L114 (47, 6) -> (53, 6)
  line L115 (53, 6) -> (57, 2)
  line L116 (57, 2) -> (53, 2)
  line L117 (53, 2) -> (53, 0)
  line L118 (53, 0) -> (67, 0)
  line L119 (67, 0) -> (67, 2)
  line L120 (67, 2) -> (63, 2)
  line L121 (63, 2) -> (67, 6)
  line L122 (67, 6) -> (73, 6)
  line L123 (73, 6) -> (77, 2)
  line L124 (77, 2) -> (73, 2)
  line L125 (73, 2) -> (73, 0)
  line L126 (73, 0) -> (87, 0)
  line L127 (87, 0) -> (87, 2)
  line L128 (87, 2) -> (83, 2)
  line L129 (83, 2) -> (87, 6)
  line L130 (87, 6) -> (93, 6)
  line L131 (93, 6) -> (97, 2)
  line L132 (97, 2) -> (93, 2)
  line L133 (93, 2) -> (93, 0)
  line L134 (93, 0) -> (100, 0)
  line L135 (100, 0) -> (100, 7)
  circle A4 centre (10, 10) radius 2.5
  line L136 (18, 13) -> (22, 13)
  line L137 (22, 13) -> (22, 17)
  line L138 (22, 17) -> (26, 13)
  line L139 (26, 13) -> (26, 7)
  line L140 (26, 7) -> (22, 3)
  line L141 (22, 3) -> (22, 7)
  line L142 (22, 7) -> (18, 7)
  line L143 (18, 7) -> (18, 3)
  line L144 (18, 3) -> (14, 7)
  line L145 (14, 7) -> (14, 13)
  line L146 (14, 13) -> (18, 17)
  line L147 (18, 17) -> (18, 13)
  line L148 (18, 17) -> (82, 17)
  line L149 (82, 3) -> (18, 3)
  constraint coincident L146.end L147.start
  constraint coincident L1.end L2.start
  constraint coincident L4.end L5.start
  constraint coincident L143.end L144.start
extrude "Extrude3''" cut sketch "Sketch3 (2)" against normal through all contours L0 L1 L11 L148 | L5 L6 L7 L149 | L12 L13 L23 L148 | L17 L18 L19 L149 | L24 L25 L35 L148 | L29 L30 L31 L149 | L136 L137 L147 L148 | L141 L142 L143 L149 bodies 5 in component "ProfileBase"
sketch "Sketch1 (5)" plane through (0, 0, 0) normal (0, 1, 0) x (1, 0, 0) in component "PVC"
  circle A0 centre (0, 0) radius 9.1
  circle A1 centre (0, 0) radius 11
  dimension "d81" = 18.2
  dimension "d82" = 22
  constraint coincident A0.centre A1.centre
  constraint concentric A0 A1
  measures "d81" diameter of A0
  measures "d82" diameter of A1
extrude "Extrude1''''" add sketch "Sketch1 (5)" against normal blind 85 separate body makes body 6 in component "PVC"
sketch "Sketch1 (6)" plane through (0, 0, 0) normal (0, 1, 0) x (1, 0, 0) in component "Bearing6804-zz-C3"
  circle A0 centre (0, 0) radius 10
  circle A1 centre (0, 0) radius 16
  dimension "d81_1" = 20
  dimension "d82_1" = 32
  constraint coincident A0.centre A1.centre
  constraint concentric A0 A1
  measures "d81_1" diameter of A0
  measures "d82_1" diameter of A1
extrude "Extrude1'''''" add sketch "Sketch1 (6)" against normal blind 7 separate body makes body 7 in component "Bearing6804-zz-C3"
component "ProfileBase" placed x (1, 0, 0) y (0, 1, 0) z (0, 0, 1) at (0, 0, 0)
component "conveyerarm v2" placed x (1, 0, 0) y (0, 1, 0) z (0, 0, 1) at (163.8256, -6.1847, -74.8631)
component "ConveyerLeg1 v3" placed x (1, 0, 0) y (0, 1, 0) z (0, 0, 1) at (189.9371, 101.1598, 13.4761)
component "CONVEYERROLLERv2 v4" placed x (1, 0, 0) y (0, 1, 0) z (0, 0, 1) at (6.7491, -74.5512, -71.8534)
component "PVC" placed x (1, 0, 0) y (0, 1, 0) z (0, 0, 1) at (-41.1686, -133.7151, -106.3935)
component "Bearing6804-zz-C3" placed x (1, 0, 0) y (0, 1, 0) z (0, 0, 1) at (-54.8449, -103.3884, -72.5511)
component "ConveyerLeg1 v3" placed x (1, 0, 0) y (0, 1, 0) z (0, 0, 1) at (217.9201, 132.429, 72.8121)
component "CONVEYERROLLERv2 v4" placed x (1, 0, 0) y (0, 1, 0) z (0, 0, 1) at (36.7491, -74.5512, -71.8534)
component "CONVEYERROLLERv2 v4" placed x (1, 0, 0) y (0, 1, 0) z (0, 0, 1) at (76.7491, -74.5512, -71.8534)
component "CONVEYERROLLERv2 v4" placed x (1, 0, 0) y (0, 1, 0) z (0, 0, 1) at (116.7491, -74.5512, -71.8534)
component "Bearing6804-zz-C3" placed x (1, 0, 0) y (0, 1, 0) z (0, 0, 1) at (-4.8449, -103.3884, -72.5511)
component "Bearing6804-zz-C3" placed x (1, 0, 0) y (0, 1, 0) z (0, 0, 1) at (45.1551, -103.3884, -72.5511)
component "Bearing6804-zz-C3" placed x (1, 0, 0) y (0, 1, 0) z (0, 0, 1) at (85.1551, -103.3884, -72.5511)
component "conveyerarm v2" placed x (1, 0, 0) y (0, 1, 0) z (0, 0, 1) at (163.8256, -86.1847, -74.8631)
component "conveyerarm v2" placed x (1, 0, 0) y (0, 1, 0) z (0, 0, 1) at (163.8256, 63.8153, -74.8631)
component "conveyerarm v2" placed x (1, 0, 0) y (0, 1, 0) z (0, 0, 1) at (163.8256, -156.1847, -74.8631)
component "PVC" placed x (1, 0, 0) y (0, 1, 0) z (0, 0, 1) at (18.8314, -133.7151, -106.3935)
component "ConveyerLeg1 v3" placed x (1, 0, 0) y (0, 1, 0) z (0, 0, 1) at (217.9201, 202.429, 72.8121)
component "ConveyerLeg1 v3" placed x (1, 0, 0) y (0, 1, 0) z (0, 0, 1) at (217.9201, 272.429, 72.8121)
